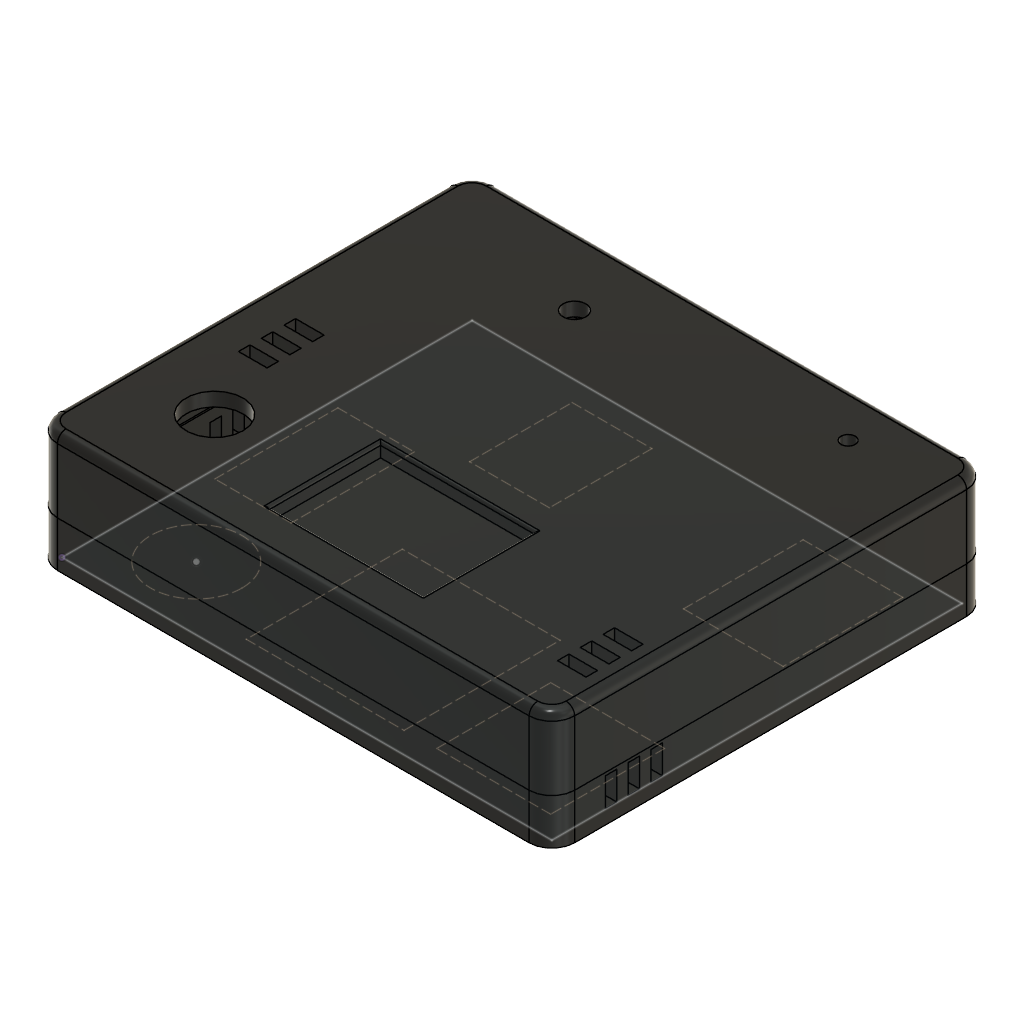
omnisensor_enclosure (Autodesk Fusion 360 design; units mm, degrees)
part number: 2026-09-06-11-30-26-147
Autodesk Fusion 360 part; units mm, degrees
sketch "Schizzo2" plane through (0, 0, 0) normal (0, 0, 1) x (1, 0, 0)
  line L0 (0, 0) -> (86, 0)
  line L1 (86, 0) -> (86, 72)
  line L2 (86, 72) -> (0, 72)
  line L3 (0, 72) -> (0, 0)
  line L4 (28.626, 3.7267) -> (56.326, 3.7267) construction
  line L5 (56.326, 3.7267) -> (56.326, 31.1267) construction
  line L6 (56.326, 31.1267) -> (28.626, 31.1267) construction
  line L7 (28.626, 31.1267) -> (28.626, 3.7267) construction
  circle A0 centre (12.4612, 11.1228) radius 8 construction
  line L8 (21.2395, 68.3222) -> (35.2395, 68.3222) construction
  line L9 (35.2395, 68.3222) -> (35.2395, 50.3222) construction
  line L10 (35.2395, 50.3222) -> (21.2395, 50.3222) construction
  line L11 (21.2395, 50.3222) -> (21.2395, 68.3222) construction
  line L12 (61.9433, 23.8505) -> (81.9433, 23.8505) construction
  line L13 (81.9433, 23.8505) -> (81.9433, 3.8505) construction
  line L14 (81.9433, 3.8505) -> (61.9433, 3.8505) construction
  line L15 (61.9433, 3.8505) -> (61.9433, 23.8505) construction
  line L16 (62.3787, 67.7242) -> (79.8787, 67.7242) construction
  line L17 (79.8787, 67.7242) -> (79.8787, 46.7242) construction
  line L18 (79.8787, 46.7242) -> (62.3787, 46.7242) construction
  line L19 (62.3787, 46.7242) -> (62.3787, 67.7242) construction
  line L20 (1.4882, 46.9493) -> (14.8882, 46.9493) construction
  line L21 (14.8882, 46.9493) -> (14.8882, 25.3493) construction
  line L22 (14.8882, 25.3493) -> (1.4882, 25.3493) construction
  line L23 (1.4882, 25.3493) -> (1.4882, 46.9493) construction
  dimension "d12" = 86
  dimension "d13" = 72
  dimension "d14" = 27.7
  dimension "d15" = 27.4
  dimension "d16" = 16
  dimension "d17" = 14
  dimension "d18" = 18
  dimension "d19" = 20
  dimension "d20" = 20
  dimension "d21" = 17.5
  dimension "d22" = 21
  dimension "d23" = 13.4
  dimension "d24" = 21.6
  constraint horizontal L0
  constraint vertical L1
  constraint horizontal L2
  constraint vertical L3
  constraint coincident L0.start L3.end
  constraint horizontal L4
  constraint vertical L5
  constraint horizontal L6
  constraint vertical L7
  constraint horizontal L8
  constraint vertical L9
  constraint horizontal L10
  constraint vertical L11
  constraint horizontal L12
  constraint vertical L13
  constraint horizontal L14
  constraint vertical L15
  constraint horizontal L16
  constraint vertical L17
  constraint horizontal L18
  constraint vertical L19
  constraint horizontal L20
  constraint vertical L21
  constraint horizontal L22
  constraint vertical L23
  measures "d12" distance of L0.start L0.end
  measures "d13" distance of L0.start L2.end
  measures "d14" distance of L4.start L4.end
  measures "d15" distance of L4.start L6.end
  measures "d16" diameter of A0
  measures "d17" distance of L8.start L8.end
  measures "d18" distance of L8.start L10.end
  measures "d19" distance of L12.start L12.end
  measures "d20" distance of L12.start L14.end
  measures "d21" distance of L16.start L16.end
  measures "d22" distance of L16.start L18.end
  measures "d23" distance of L20.start L20.end
  measures "d24" distance of L20.start L22.end
sketch "Sketch10" plane through (0, 0, 0) normal (0, 0, 1) x (1, 0, 0)
  line L0 (84.4004, 74.4002) -> (1.6004, 74.4002)
  line L1 (-2.3996, 70.4002) -> (-2.3996, 1.6002)
  line L2 (1.6004, -2.3998) -> (84.4004, -2.3998)
  line L3 (88.4004, 1.6002) -> (88.4004, 70.4002)
  line L4 (88.4004, 74.4002) -> (-2.3996, -2.3998) construction
  line L5 (-2.3996, 74.4002) -> (88.4004, -2.3998) construction
  arc A0 (1.6004, 74.4002) -> (-2.3996, 70.4002) centre (1.6004, 70.4002) ccw
  arc A1 (88.4004, 70.4002) -> (84.4004, 74.4002) centre (84.4004, 70.4002) ccw
  arc A2 (-2.3996, 1.6002) -> (1.6004, -2.3998) centre (1.6004, 1.6002) ccw
  arc A3 (84.4004, -2.3998) -> (88.4004, 1.6002) centre (84.4004, 1.6002) ccw
  point P0 (43.0004, 36.0002)
  dimension "d49" = 90.8
  dimension "d50" = 76.8
  dimension "d51" = 4
  dimension "d52" = 4
  dimension "d53" = 4
  dimension "d54" = 4
  constraint horizontal L0
  constraint perpendicular L0 L1
  constraint parallel L0 L2
  constraint parallel L1 L3
  constraint coincident L4 P0
  constraint coincident L5 P0
  constraint coincident L5.start L1
  constraint coincident L5.start L0
  constraint tangent L1 A0
  constraint tangent L0 A0
  constraint coincident L4.start L0
  constraint coincident L4.start L3
  constraint tangent L0 A1
  constraint tangent L3 A1
  constraint coincident L4.end L1
  constraint coincident L4.end L2
  constraint tangent L1 A2
  constraint tangent L2 A2
  constraint coincident L5.end L3
  constraint coincident L5.end L2
  constraint tangent L3 A3
  constraint tangent L2 A3
  measures "d49" distance of L4.end L5.end
  measures "d50" distance of L5.start L4.end
  measures "d51" radius of A0
  measures "d52" radius of A1
  measures "d53" radius of A2
  measures "d54" radius of A3
extrude "Extrude3" add sketch "Sketch10" along normal blind 20.8 makes body 1
ref_plane "WorkPlane2" through (43, 36, 8) normal (0, 0, 1) x (1, 0, 0)
split "Split2" by plane through (43, 36, 8) normal (0, 0, 1) bodies 1 makes body 2 at (29.2004, 48.8002, 20.8)
shell "Shell3" thickness 2.4 removed faces 1 at (29.2004, 48.8002, 8) on bodies 1
shell "Shell4" thickness 2.4 removed faces 1 at (29.2004, 48.8002, 8) on bodies 2
sketch "Sketch11" plane through (0, 0, 8) normal (0, 0, 1) x (-1, 0, 0)
  line L0 (-1.6004, -72.0002) -> (-84.4004, -72.0002)
  arc A0 (-86.0004, -70.4002) -> (-84.4004, -72.0002) centre (-84.4004, -70.4002) ccw
  line L1 (-86.0004, -70.4002) -> (-86.0004, -1.6002)
  arc A1 (-84.4004, -0.0002) -> (-86.0004, -1.6002) centre (-84.4004, -1.6002) ccw
  line L2 (-84.4004, -0.0002) -> (-1.6004, -0.0002)
  arc A2 (-0.0004, -1.6002) -> (-1.6004, -0.0002) centre (-1.6004, -1.6002) ccw
  line L3 (-0.0004, -1.6002) -> (-0.0004, -70.4002)
  arc A3 (-1.6004, -72.0002) -> (-0.0004, -70.4002) centre (-1.6004, -70.4002) ccw
  line L4 (-1.6004, 2.3998) -> (-84.4004, 2.3998)
  arc A4 (-84.4004, 2.3998) -> (-88.4004, -1.6002) centre (-84.4004, -1.6002) ccw
  line L5 (-88.4004, -1.6002) -> (-88.4004, -70.4002)
  arc A5 (-88.4004, -70.4002) -> (-84.4004, -74.4002) centre (-84.4004, -70.4002) ccw
  line L6 (-84.4004, -74.4002) -> (-1.6004, -74.4002)
  arc A6 (-1.6004, -74.4002) -> (2.3996, -70.4002) centre (-1.6004, -70.4002) ccw
  line L7 (2.3996, -70.4002) -> (2.3996, -1.6002)
  arc A7 (2.3996, -1.6002) -> (-1.6004, 2.3998) centre (-1.6004, -1.6002) ccw
  line L8 (-84.4004, -73.2002) -> (-1.6004, -73.2002)
  arc A8 (-1.6004, -73.2002) -> (1.1996, -70.4002) centre (-1.6004, -70.4002) ccw
  line L9 (1.1996, -70.4002) -> (1.1996, -1.6002)
  arc A9 (1.1996, -1.6002) -> (-1.6004, 1.1998) centre (-1.6004, -1.6002) ccw
  line L10 (-1.6004, 1.1998) -> (-84.4004, 1.1998)
  arc A10 (-84.4004, 1.1998) -> (-87.2004, -1.6002) centre (-84.4004, -1.6002) ccw
  line L11 (-87.2004, -1.6002) -> (-87.2004, -70.4002)
  arc A11 (-87.2004, -70.4002) -> (-84.4004, -73.2002) centre (-84.4004, -70.4002) ccw
extrude "Extrude4" add sketch "Sketch11" along normal blind 1.5 contours L8 A8 L9 A9 L10 A10 L11 A11 bodies 1
chamfer "Chamfer1" distance 0.3 angle 45 8 edges at (87.2004, 36.0002, 9.5) (86.3803, 72.3801, 9.5) (43.0004, 73.2002, 9.5) (-0.3795, 72.3801, 9.5) (-1.1996, 36.0002, 9.5) (-0.3795, -0.3797, 9.5) (43.0004, -1.1998, 9.5) (86.3803, -0.3797, 9.5) tangent chain off on bodies 1
sketch "Sketch12" plane through (0, 0, 8) normal (0, 0, -1) x (1, 0, 0)
  line L0 (84.4004, -72.0002) -> (1.6004, -72.0002)
  arc A0 (0.0004, -70.4002) -> (1.6004, -72.0002) centre (1.6004, -70.4002) ccw
  line L1 (0.0004, -70.4002) -> (0.0004, -1.6002)
  arc A1 (1.6004, -0.0002) -> (0.0004, -1.6002) centre (1.6004, -1.6002) ccw
  line L2 (1.6004, -0.0002) -> (84.4004, -0.0002)
  arc A2 (86.0004, -1.6002) -> (84.4004, -0.0002) centre (84.4004, -1.6002) ccw
  line L3 (86.0004, -1.6002) -> (86.0004, -70.4002)
  arc A3 (84.4004, -72.0002) -> (86.0004, -70.4002) centre (84.4004, -70.4002) ccw
  line L4 (84.4004, 2.3998) -> (1.6004, 2.3998)
  arc A4 (1.6004, 2.3998) -> (-2.3996, -1.6002) centre (1.6004, -1.6002) ccw
  line L5 (-2.3996, -1.6002) -> (-2.3996, -70.4002)
  arc A5 (-2.3996, -70.4002) -> (1.6004, -74.4002) centre (1.6004, -70.4002) ccw
  line L6 (1.6004, -74.4002) -> (84.4004, -74.4002)
  arc A6 (84.4004, -74.4002) -> (88.4004, -70.4002) centre (84.4004, -70.4002) ccw
  line L7 (88.4004, -70.4002) -> (88.4004, -1.6002)
  arc A7 (88.4004, -1.6002) -> (84.4004, 2.3998) centre (84.4004, -1.6002) ccw
  line L8 (1.6004, -73.4502) -> (84.4004, -73.4502)
  arc A8 (84.4004, -73.4502) -> (87.4504, -70.4002) centre (84.4004, -70.4002) ccw
  line L9 (87.4504, -70.4002) -> (87.4504, -1.6002)
  arc A9 (87.4504, -1.6002) -> (84.4004, 1.4498) centre (84.4004, -1.6002) ccw
  line L10 (84.4004, 1.4498) -> (1.6004, 1.4498)
  arc A10 (1.6004, 1.4498) -> (-1.4496, -1.6002) centre (1.6004, -1.6002) ccw
  line L11 (-1.4496, -1.6002) -> (-1.4496, -70.4002)
  arc A11 (-1.4496, -70.4002) -> (1.6004, -73.4502) centre (1.6004, -70.4002) ccw
extrude "Extrude5" cut sketch "Sketch12" against normal blind 1.8 contours L8 A8 L9 A9 L10 A10 L11 A11 bodies 2
sketch "Sketch15" plane through (0, 0, 20.8) normal (0, 0, 1) x (-1, 0, 0)
  arc A0 (-84.4004, 2.3998) -> (-88.4004, -1.6002) centre (-84.4004, -1.6002) ccw
  line L0 (-88.4004, -1.6002) -> (-88.4004, -70.4002)
  arc A1 (-88.4004, -70.4002) -> (-84.4004, -74.4002) centre (-84.4004, -70.4002) ccw
  line L1 (-84.4004, -74.4002) -> (-1.6004, -74.4002)
  arc A2 (-1.6004, -74.4002) -> (2.3996, -70.4002) centre (-1.6004, -70.4002) ccw
  line L2 (2.3996, -70.4002) -> (2.3996, -1.6002)
  arc A3 (2.3996, -1.6002) -> (-1.6004, 2.3998) centre (-1.6004, -1.6002) ccw
  line L3 (-1.6004, 2.3998) -> (-84.4004, 2.3998)
  line L4 (-58.2335, -5.1871) -> (-31.2335, -5.1871)
  line L5 (-31.2335, -5.1871) -> (-31.2335, -24.6871)
  line L6 (-31.2335, -24.6871) -> (-58.2335, -24.6871)
  line L7 (-58.2335, -24.6871) -> (-58.2335, -5.1871)
  line L8 (-58.2335, -5.1871) -> (-31.2335, -24.6871) construction
  line L9 (-31.2335, -5.1871) -> (-58.2335, -24.6871) construction
  circle A4 centre (-12.4506, -14.33) radius 5
  circle A5 centre (-28.2279, -61.7393) radius 2
  circle A6 centre (-72, -66) radius 1.25
  point P0 (-44.7335, -14.9371)
  dimension "d77" = 27
  dimension "d78" = 19.5
  dimension "d79" = 10
  dimension "d80" = 4
  dimension "d81" = 2.5
  constraint horizontal L4
  constraint perpendicular L4 L5
  constraint parallel L4 L6
  constraint parallel L5 L7
  constraint coincident L8 P0
  constraint coincident L9 P0
  measures "d77" distance of L5.end L6.end
  measures "d78" distance of L4.end L5.end
  measures "d79" diameter of A4
  measures "d80" diameter of A5
  measures "d81" diameter of A6
extrude "Extrude6" cut sketch "Sketch15" against normal blind 5 contours L4 L5 L6 L7 | A4 | A5 | A6 bodies 2
sketch "Sketch16" plane through (0, 74.4002, 0) normal (0, 1, 0) x (-1, 0, 0)
  line L0 (-1.6004, 8) -> (-84.4004, 8)
  line L1 (-84.4004, 8) -> (-84.4004, 0)
  line L2 (-84.4004, 0) -> (-1.6004, 0)
  line L3 (-1.6004, 0) -> (-1.6004, 8)
  line L4 (-65.5175, 2.4288) -> (-75.0175, 2.4288)
  line L5 (-75.0175, 2.4288) -> (-75.0175, 6.2288)
  line L6 (-75.0175, 6.2288) -> (-65.5175, 6.2288)
  line L7 (-65.5175, 6.2288) -> (-65.5175, 2.4288)
  line L8 (-65.5175, 2.4288) -> (-75.0175, 6.2288) construction
  line L9 (-75.0175, 2.4288) -> (-65.5175, 6.2288) construction
  point P0 (-70.2675, 4.3288)
  dimension "d84" = 9.5
  dimension "d85" = 3.8
  constraint horizontal L4
  constraint perpendicular L4 L5
  constraint parallel L4 L6
  constraint parallel L5 L7
  constraint coincident L8 P0
  constraint coincident L9 P0
  measures "d84" distance of L5.end L6.end
  measures "d85" distance of L4.end L5.end
extrude "Extrude7" cut sketch "Sketch16" against normal blind 5 contours L4 L5 L6 L7 bodies 1
sketch "Sketch17" plane through (-2.3996, 0, 0) normal (-1, 0, 0) x (0, -1, 0)
  line L0 (-1.6002, 8) -> (-70.4002, 8)
  line L1 (-70.4002, 8) -> (-70.4002, 0)
  line L2 (-70.4002, 0) -> (-1.6002, 0)
  line L3 (-1.6002, 0) -> (-1.6002, 8)
  line L4 (-34, 2.5) -> (-36, 2.5)
  line L5 (-36, 2.5) -> (-36, 7.5)
  line L6 (-36, 7.5) -> (-34, 7.5)
  line L7 (-34, 7.5) -> (-34, 2.5)
  line L8 (-34, 2.5) -> (-36, 7.5) construction
  line L9 (-36, 2.5) -> (-34, 7.5) construction
  line L10 (-30, 2.5) -> (-32, 2.5)
  line L11 (-32, 2.5) -> (-32, 7.5)
  line L12 (-32, 7.5) -> (-30, 7.5)
  line L13 (-30, 7.5) -> (-30, 2.5)
  line L14 (-30, 2.5) -> (-32, 7.5) construction
  line L15 (-32, 2.5) -> (-30, 7.5) construction
  line L16 (-26, 2.5) -> (-28, 2.5)
  line L17 (-28, 2.5) -> (-28, 7.5)
  line L18 (-28, 7.5) -> (-26, 7.5)
  line L19 (-26, 7.5) -> (-26, 2.5)
  line L20 (-26, 2.5) -> (-28, 7.5) construction
  line L21 (-28, 2.5) -> (-26, 7.5) construction
  point P0 (-35, 5)
  point P1 (-31, 5)
  point P2 (-27, 5)
  dimension "d88" = 2
  dimension "d89" = 5
  dimension "d90" = 2
  dimension "d91" = 5
  dimension "d92" = 2
  constraint horizontal L4
  constraint perpendicular L4 L5
  constraint parallel L4 L6
  constraint parallel L5 L7
  constraint coincident L8 P0
  constraint coincident L9 P0
  constraint horizontal L10
  constraint perpendicular L10 L11
  constraint parallel L10 L12
  constraint parallel L11 L13
  constraint coincident L14 P1
  constraint coincident L15 P1
  constraint horizontal L16
  constraint perpendicular L16 L17
  constraint parallel L16 L18
  constraint parallel L17 L19
  constraint coincident L20 P2
  constraint coincident L21 P2
  measures "d88" distance of L5.end L6.end
  measures "d89" distance of L4.end L5.end
  measures "d90" distance of L11.end L12.end
  measures "d91" distance of L10.end L11.end
  measures "d92" distance of L17.end L18.end
extrude "Extrude8" cut sketch "Sketch17" against normal blind 5 contours L4 L5 L6 L7 | L10 L11 L12 L13 | L16 L17 L18 L19 bodies 1
sketch "Sketch18" plane through (88.4004, 0, 0) normal (1, 0, 0) x (0, 1, 0)
  line L0 (70.4002, 8) -> (1.6002, 8)
  line L1 (1.6002, 8) -> (1.6002, 0)
  line L2 (1.6002, 0) -> (70.4002, 0)
  line L3 (70.4002, 0) -> (70.4002, 8)
  line L4 (9, 7.5) -> (7, 7.5)
  line L5 (7, 7.5) -> (7, 2.5)
  line L6 (7, 2.5) -> (9, 2.5)
  line L7 (9, 2.5) -> (9, 7.5)
  line L8 (9, 7.5) -> (7, 2.5) construction
  line L9 (7, 7.5) -> (9, 2.5) construction
  line L10 (11, 7.5) -> (13, 7.5)
  line L11 (13, 7.5) -> (13, 2.5)
  line L12 (13, 2.5) -> (11, 2.5)
  line L13 (11, 2.5) -> (11, 7.5)
  line L14 (15, 7.5) -> (17, 7.5)
  line L15 (17, 7.5) -> (17, 2.5)
  line L16 (17, 2.5) -> (15, 2.5)
  line L17 (15, 2.5) -> (15, 7.5)
  point P0 (8, 5)
  dimension "d95" = 2
  dimension "d96" = 5
  constraint horizontal L4
  constraint perpendicular L4 L5
  constraint parallel L4 L6
  constraint parallel L5 L7
  constraint coincident L8 P0
  constraint coincident L9 P0
  constraint horizontal L10
  constraint vertical L11
  constraint horizontal L12
  constraint vertical L13
  constraint horizontal L14
  constraint vertical L15
  constraint horizontal L16
  constraint vertical L17
  measures "d95" distance of L5.end L6.end
  measures "d96" distance of L4.end L5.end
extrude "Extrude9" cut sketch "Sketch18" against normal blind 5 contours L4 L5 L6 L7 | L10 L11 L12 L13 | L14 L15 L16 L17 bodies 1
sketch "Sketch19" plane through (0, 0, 20.8) normal (0, 0, 1) x (-1, 0, 0)
  circle A0 centre (-72, -66) radius 1.25
  line L0 (-31.2335, -5.1871) -> (-31.2335, -24.6871)
  line L1 (-31.2335, -24.6871) -> (-58.2335, -24.6871)
  line L2 (-58.2335, -24.6871) -> (-58.2335, -5.1871)
  line L3 (-58.2335, -5.1871) -> (-31.2335, -5.1871)
  circle A1 centre (-28.2279, -61.7393) radius 2
  circle A2 centre (-12.4506, -14.33) radius 5
  arc A3 (-84.4004, 2.3998) -> (-88.4004, -1.6002) centre (-84.4004, -1.6002) ccw
  line L4 (-88.4004, -1.6002) -> (-88.4004, -70.4002)
  arc A4 (-88.4004, -70.4002) -> (-84.4004, -74.4002) centre (-84.4004, -70.4002) ccw
  line L5 (-84.4004, -74.4002) -> (-1.6004, -74.4002)
  arc A5 (-1.6004, -74.4002) -> (2.3996, -70.4002) centre (-1.6004, -70.4002) ccw
  line L6 (2.3996, -70.4002) -> (2.3996, -1.6002)
  arc A6 (2.3996, -1.6002) -> (-1.6004, 2.3998) centre (-1.6004, -1.6002) ccw
  line L7 (-1.6004, 2.3998) -> (-84.4004, 2.3998)
  line L8 (-85, -7) -> (-80, -7)
  line L9 (-80, -7) -> (-80, -9)
  line L10 (-80, -9) -> (-85, -9)
  line L11 (-85, -9) -> (-85, -7)
  line L12 (-85, -11) -> (-80, -11)
  line L13 (-80, -11) -> (-80, -13)
  line L14 (-80, -13) -> (-85, -13)
  line L15 (-85, -13) -> (-85, -11)
  line L16 (-85, -15) -> (-80, -15)
  line L17 (-80, -15) -> (-80, -17)
  line L18 (-80, -17) -> (-85, -17)
  line L19 (-85, -17) -> (-85, -15)
  line L20 (-5, -32) -> (-10, -32)
  line L21 (-10, -32) -> (-10, -30)
  line L22 (-10, -30) -> (-5, -30)
  line L23 (-5, -30) -> (-5, -32)
  line L24 (-5, -28) -> (-10, -28)
  line L25 (-10, -28) -> (-10, -26)
  line L26 (-10, -26) -> (-5, -26)
  line L27 (-5, -26) -> (-5, -28)
  line L28 (-5, -34) -> (-10, -34)
  line L29 (-10, -34) -> (-10, -36)
  line L30 (-10, -36) -> (-5, -36)
  line L31 (-5, -36) -> (-5, -34)
  constraint horizontal L8
  constraint vertical L9
  constraint horizontal L10
  constraint vertical L11
  constraint horizontal L12
  constraint vertical L13
  constraint horizontal L14
  constraint vertical L15
  constraint horizontal L16
  constraint vertical L17
  constraint horizontal L18
  constraint vertical L19
  constraint horizontal L20
  constraint vertical L21
  constraint horizontal L22
  constraint vertical L23
  constraint horizontal L24
  constraint vertical L25
  constraint horizontal L26
  constraint vertical L27
  constraint horizontal L28
  constraint vertical L29
  constraint horizontal L30
  constraint vertical L31
extrude "Extrude10" cut sketch "Sketch19" against normal blind 5 contours L8 L9 L10 L11 | L12 L13 L14 L15 | L16 L17 L18 L19 | L20 L21 L22 L23 | L24 L25 L26 L27 | L28 L29 L30 L31 bodies 2
fillet "Fillet1" radius 1.5 8 edges at (43.0004, 74.4002, 20.8) (-1.2281, 73.2287, 20.8) (-2.3996, 36.0002, 20.8) (-1.2281, -1.2282, 20.8) (43.0004, -2.3998, 20.8) (87.2288, -1.2282, 20.8) (88.4004, 36.0002, 20.8) (87.2288, 73.2287, 20.8) on bodies 2
fillet "Fillet2" radius 0.5 4 edges at (44.7335, 24.6871, 20.8) (58.2335, 14.9371, 20.8) (44.7335, 5.1871, 20.8) (31.2335, 14.9371, 20.8) on bodies 2
equation "wall_thick = 2.4 mm"
equation "tol_xy = 0.3 mm"
equation "hole_comp = 0.2 mm"
equation "vert_clearance = 0.5 mm"
equation "cavity_depth = 16 mm"
equation "lip_width = 1.2 mm"
equation "lip_height = 1.5 mm"
equation "lip_tol = 0.25 mm"
equation "instert_dia = 4.2 mm"
equation "insert_depth = 5 mm"
equation "m3_loose_dia = 3.4 mm"
equation "d49 = 86 mm + 2 * wall_thick"
equation "d50 = 72 mm + 2 * wall_thick"
equation "d55 = cavity_depth + 2 * wall_thick"
equation "d57 = cavity_depth / 2"
equation "d59 = wall_thick"
equation "d60 = wall_thick"
equation "d61 = -lip_width"
equation "d62 = lip_height"
equation "d65 = -( lip_width - lip_tol )"
equation "d66 = -( lip_height + 0.3 mm )"
named bodies: "Rear_Shell_Body", "Front_Shell_Body"
